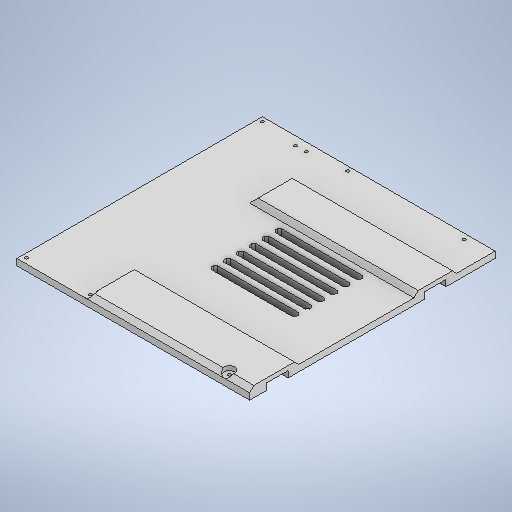
# Autodesk Inventor part: Honigschleuder_Steuerung_Netzteil_Deckel
Saved by Autodesk Inventor 2025 (Build 290162010, 162A)
## iProperties
Created: 2025-12-07
Part Number: Honigschleuder_Steuerung_Netzteil_Deckel
Material: Generisch
Document SubType Name: Modeling
Designer: max-h
Density: 1 g/cm^3
Appearance: Vorgabe
Author: max-h
Autodesk Inventor part; units mm, degrees
ref_plane "YZ Plane" through (0, 0, 0) normal (1, 0, 0) x (0, 1, 0)
ref_plane "XZ Plane" through (0, 0, 0) normal (0, 1, 0) x (-1, 0, 0)
ref_plane "XY Plane" through (0, 0, 0) normal (0, 0, 1) x (1, 0, 0)
sketch "Skizze1" plane through (0, 0, 0) normal (0, 1, 0) x (-1, 0, 0)
  line L0 (0, 0) -> (-109, 0)
  line L1 (-109, 0) -> (-109, -8)
  line L2 (-109, -115) -> (0, -115)
  line L3 (0, -115) -> (0, 0)
  line L4 (-2, -2.5) -> (-97, -2.5) construction
  line L5 (-97, -2.5) -> (-97, -113) construction
  line L6 (-97, -113) -> (-2, -113) construction
  line L7 (-2, -113) -> (-2, -2.5) construction
  circle A0 centre (-2, -2.5) radius 0.7
  circle A1 centre (-2, -113) radius 0.7
  circle A2 centre (-42, -113) radius 0.7
  circle A3 centre (-32, -2.5) radius 0.7
  circle A4 centre (-97, -2.5) radius 0.7
  line L8 (-37, -8) -> (-109, -8)
  line L9 (-109, -18) -> (-37, -18)
  line L10 (-37, -18) -> (-37, -8)
  line L11 (-37, -92) -> (-109, -92)
  line L12 (-109, -82) -> (-37, -82)
  line L13 (-37, -82) -> (-37, -92)
  line L14 (-109, -92) -> (-109, -115)
  line L15 (-109, -82) -> (-109, -92) construction
  line L16 (-109, -18) -> (-109, -82)
  line L17 (-109, -8) -> (-109, -18) construction
  circle A5 centre (-97, -112.5) radius 0.7
  dimension "d0" = 109
  dimension "d1" = 115
  dimension "d2" = 2
  dimension "d3" = 1.4
  dimension "d4" = 30
  dimension "d5" = 40
  dimension "d14" = 10
  dimension "d15" = 72
  dimension "d16" = 8
  dimension "d17" = 23
  dimension "d30" = 2.5
  dimension "d49" = 65
  dimension "d50" = 0.5
  constraints: 36 end point, 10 parallel, 8 perpendicular, 6 centre point, 5 equal radius, 4 coincident, 3 horizontal, 3 point on line, 2 equal length, 1 other
  measures "d0" distance of L0.start L0.end
  measures "d1" distance of L2.end L0.start
  measures "d2" distance between parallel lines of L3 L7
  measures "d3" diameter of A0
  measures "d4" distance from line of L7 A3.centre
  measures "d5" distance from line of L7 A2.centre
  measures "d14" distance of L1.end L9.start
  measures "d15" distance of L12.start L12.end
  measures "d16" distance between parallel lines of L0 L8
  measures "d17" distance between parallel lines of L2 L11
  measures "d30" distance between parallel lines of L0 L4
  measures "d49" distance of A4.centre A3.centre
  measures "d50" distance of L5.end A5.centre
extrude "Extrusion1" add sketch "Skizze1" along normal blind 3
sketch "Skizze3" plane through (0, 3, 0) normal (0, 1, 0) x (1, 0, 0)
  line L0 (0, 0) -> (109, 0) projected
  line L1 (109, 0) -> (34, 0)
  line L2 (34, 0) -> (34, 21)
  line L3 (34, 21) -> (109, 21)
  line L4 (109, 21) -> (109, 0)
  line L5 (37, 8) -> (37, 18) projected
  line L6 (37, 18) -> (109, 18) projected
  circle A0 centre (32, 2.5) radius 0.7 projected
  circle A1 centre (97, 2.5) radius 0.7 projected
  line L7 (109, 92) -> (109, 115) projected
  line L8 (34, 79) -> (109, 79)
  line L9 (109, 79) -> (109, 95)
  line L10 (109, 95) -> (34, 95)
  line L11 (34, 95) -> (34, 79)
  line L12 (109, 82) -> (37, 82) projected
  line L13 (37, 92) -> (109, 92) projected
  line L14 (37, 82) -> (37, 92) projected
  point P0 (109, 95)
  point P1 (97, 2.7)
  point P2 (97, 1.3)
  dimension "d18" = 3
  dimension "d19" = 3
  dimension "d20" = 3
  dimension "d21" = 3
  dimension "d22" = 3
  constraints: 14 end point, 3 parallel, 2 horizontal, 2 perpendicular, 1 point on line, 1 vertical, 4 other
  measures "d18" distance between parallel lines of L5 L2
  measures "d19" distance between parallel lines of L6 L3
  measures "d20" distance between parallel lines of L12 L8
  measures "d21" distance between parallel lines of L13 L10
  measures "d22" distance between parallel lines of L14 L11
extrude "Extrusion2" add sketch "Skizze3" along normal blind 2 contours L2 L3 L4 L0 | A1 | L13 L14 L12 L9 L8 L11 L10 L7 | L9 L12 L14 L13
chamfer "Fasen1" distance 2 angle 45 6 edges at (71.5, 3, -21) (34, 3, -10.5) (34, 3, -87) (71.5, 3, -79) (71.5, 3, -95) (71.5, 5, 0)
sketch "Skizze5" plane through (0, 0, 0) normal (0, -1, 0) x (1, 0, 0)
  circle A0 centre (19.5, -111) radius 0.7
  circle A1 centre (24.5, -111) radius 0.7
  line L0 (17, -111) -> (27, -111) construction
  line L1 (109, -115) -> (0, -115) construction
  line L2 (0, -115) -> (0, 0) construction
  dimension "d31" = 17
  dimension "d32" = 10
  dimension "d33" = 1.4
  dimension "d34" = 4
  dimension "d35" = 5
  dimension "d36" = 2.5
  constraints: 2 centre point, 2 end point, 2 point on line, 1 equal radius, 1 parallel
  measures "d31" distance from line of L2 L0.start
  measures "d32" distance of L0.start L0.end
  measures "d33" diameter of A0
  measures "d34" distance between parallel lines of L1 L0
  measures "d35" distance of A0.centre A1.centre
  measures "d36" distance of L0.start A0.centre
extrude "Extrusion4" cut sketch "Skizze5" against normal through all
sketch "Skizze6" plane through (0, 5, 0) normal (0, 1, 0) x (1, 0, 0)
  circle A0 centre (32, 2.5) radius 0.7 projected
  circle A1 centre (32, 2.5) radius 2.5
  circle A2 centre (97, 2.5) radius 0.7 projected
  circle A3 centre (97, 2.5) radius 2.5
  point P0 (0, 0)
  point P1 (97, 2.7)
  point P2 (97, 1.3)
  dimension "d46" = 5
  constraints: 2 centre point, 2 coincident, 1 equal radius, 1 other
  measures "d46" diameter of A1
extrude "Extrusion5" cut sketch "Skizze6" against normal blind 2 contours A1 | A2 | A3
sketch "Skizze7" plane through (0, 3, 0) normal (0, 1, 0) x (1, 0, 0)
  line L0 (49, 41) -> (89, 41)
  line L1 (89, 41) -> (89, 77)
  line L2 (89, 77) -> (49, 77) construction
  line L3 (49, 77) -> (49, 41)
  circle A0 centre (97, 2.5) radius 0.7 projected
  line L4 (109, 23) -> (32, 23) projected
  line L5 (32, 77) -> (109, 77) projected
  line L6 (49, 44) -> (89, 44)
  line L7 (89, 44) -> (89, 47)
  line L8 (89, 47) -> (49, 47)
  line L9 (49, 47) -> (49, 44)
  line L10 (49, 50) -> (89, 50)
  line L11 (89, 50) -> (89, 53)
  line L12 (89, 53) -> (49, 53)
  line L13 (49, 53) -> (49, 50)
  line L14 (49, 56) -> (89, 56)
  line L15 (89, 56) -> (89, 59)
  line L16 (89, 59) -> (49, 59)
  line L17 (49, 59) -> (49, 56)
  line L18 (49, 62) -> (89, 62)
  line L19 (89, 62) -> (89, 65)
  line L20 (89, 65) -> (49, 65)
  line L21 (49, 65) -> (49, 62)
  line L22 (49, 68) -> (89, 68)
  line L23 (89, 68) -> (89, 71)
  line L24 (89, 71) -> (49, 71)
  line L25 (49, 71) -> (49, 68)
  line L26 (49, 77) -> (89, 77)
  line L27 (89, 77) -> (89, 74)
  line L28 (89, 74) -> (49, 74)
  line L29 (49, 74) -> (49, 77)
  point P0 (0, 0)
  point P1 (89, 68)
  point P2 (49, 65)
  point P3 (89, 62)
  point P4 (49, 59)
  point P5 (89, 56)
  point P6 (49, 53)
  point P7 (89, 50)
  point P8 (49, 47)
  dimension "d51" = 8
  dimension "d52" = 18
  dimension "d53" = 40
  dimension "d54" = 3
  dimension "d55" = 3
  dimension "d56" = 3
  dimension "d57" = 3
  dimension "d58" = 3
  dimension "d59" = 3
  dimension "d60" = 3
  dimension "d61" = 3
  dimension "d62" = 3
  dimension "d63" = 3
  dimension "d64" = 3
  constraints: 56 end point, 14 parallel, 11 point on line, 7 horizontal, 7 perpendicular, 1 midpoint
  measures "d51" distance from line of L1 A0.centre
  measures "d52" distance between parallel lines of L4 L0
  measures "d53" distance of L0.start L0.end
  measures "d54" distance between parallel lines of L0 L6
  measures "d55" distance between parallel lines of L6 L8
  measures "d56" distance between parallel lines of L10 L8
  measures "d57" distance between parallel lines of L12 L10
  measures "d58" distance between parallel lines of L14 L12
  measures "d59" distance between parallel lines of L16 L14
  measures "d60" distance between parallel lines of L18 L16
  measures "d61" distance between parallel lines of L20 L18
  measures "d62" distance between parallel lines of L22 L20
  measures "d63" distance between parallel lines of L24 L22
  measures "d64" distance between parallel lines of L28 L24
extrude "Extrusion6" cut sketch "Skizze7" against normal blind 10 contours L3 L6 L1 L0 | L3 L10 L1 L8 | L3 L14 L1 L12 | L3 L18 L1 L16 | L3 L22 L1 L20 | L3 L28 L1 L24
chamfer "Fasen2" distance 1 angle 45 24 edges at (49, 1.5, -41) (49, 1.5, -44) (49, 1.5, -50) (49, 1.5, -47) (49, 1.5, -53) (49, 1.5, -59) (49, 1.5, -71) (49, 1.5, -65) (49, 1.5, -62) (49, 1.5, -68) (49, 1.5, -74) (89, 1.5, -74) (89, 1.5, -68) (89, 1.5, -62) (89, 1.5, -56) (89, 1.5, -50) (89, 1.5, -44) (89, 1.5, -41) (89, 1.5, -47) (89, 1.5, -53) (89, 1.5, -59) (89, 1.5, -65) (89, 1.5, -71) (49, 1.5, -56)
